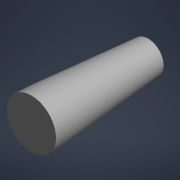
# Autodesk Inventor part: Figure
Saved by Autodesk Inventor 2021.4 (Build 254397000, 397)
## iProperties
Part Number: Figure
Material: Generic
Document SubType Name: Modeling
Designer: jo_ki
Appearance: Default
Author: jo_ki
Autodesk Inventor part; units mm, degrees
ref_plane "YZ Plane" through (0, 0, 0) normal (1, 0, 0) x (0, 1, 0)
ref_plane "XZ Plane" through (0, 0, 0) normal (0, 1, 0) x (-1, 0, 0)
ref_plane "XY Plane" through (0, 0, 0) normal (0, 0, 1) x (1, 0, 0)
sketch "Sketch1" plane through (0, 0, 0) normal (1, 0, 0) x (0, 1, 0)
  line L0 (0, -734.2857) -> (115.4555, -734.2857)
  line L1 (170, -174.2857) -> (125.4229, -725.0924)
  arc A0 (115.4555, -734.2857) -> (125.4229, -725.0924) centre (115.4555, -724.2857) ccw
  line L2 (0, -922.6226) -> (0, 382.1038) projected
  line L3 (170, -174.2857) -> (190, 65.7143)
  line L4 (190, 65.7143) -> (195, 195.7143)
  line L5 (195, 195.7143) -> (0, 195.7143)
  point P0 (0, 0)
  point P1 (124.6789, -734.2857)
  dimension "d2" = 10
  dimension "d3" = 560
  dimension "d4" = 340
  dimension "d5" = 380
  dimension "d6" = 800
  dimension "d7" = 390
  dimension "d8" = 930
  constraints: 10 end point, 4 point on line, 2 point on circle, 2 tangent, 1 centre point, 1 perpendicular
  measures "d2" radius of A0
  measures "d3" distance from line of L0 L1.start
  measures "d4" diameter of L1.start L2
  measures "d5" diameter of L3.end L2
  measures "d6" distance from line of L0 L3.end
  measures "d7" diameter of L4.end L2
  measures "d8" distance from line of L0 L4.end
revolve "Revolution1" add sketch "Sketch1" angle 360 about axis through (0, 0, -10) along (0, 0, 1)
body "Solid1"
